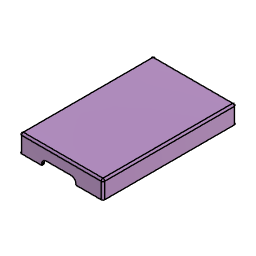
SlimCase-602030-FDM-Cover v3 (Autodesk Fusion 360 design; units mm, degrees)
Autodesk Fusion 360 part; units mm, degrees
sketch "Sketch1" plane through (0, 0, 0) normal (0, 0, 1) x (1, 0, 0)
  line L0 (11.7, 18.75) -> (-11.7, 18.75)
  line L1 (-11.7, 18.75) -> (-11.7, -18.75)
  line L2 (-11.7, -18.75) -> (11.7, -18.75)
  line L3 (11.7, -18.75) -> (11.7, 18.75)
  line L4 (11.7, 18.75) -> (-11.7, -18.75) construction
  line L5 (-11.7, 18.75) -> (11.7, -18.75) construction
  dimension "d1" = 23.4
  dimension "d2" = 37.5
  constraint horizontal L0
  constraint perpendicular L0 L1
  constraint parallel L0 L2
  constraint parallel L1 L3
  constraint coincident L4 origin
  constraint coincident L5 origin
  measures "d1" distance of L0.start L0.end
  measures "d2" distance of L0.end L1.end
extrude "Extrude1" add sketch "Sketch1" along normal blind 3.5
sketch "Sketch2" plane through (0, 0, 0) normal (0, 0, -1) x (1, 0, 0)
  line L0 (11.7, -18.75) -> (11.7, 18.75)
  line L1 (11.7, 18.75) -> (-11.7, 18.75)
  line L2 (-11.7, 18.75) -> (-11.7, -18.75)
  line L3 (-11.7, -18.75) -> (11.7, -18.75)
  line L4 (-10.1, -17.15) -> (10.1, -17.15)
  line L5 (10.1, -17.15) -> (10.1, 17.15)
  line L6 (10.1, 17.15) -> (-10.1, 17.15)
  line L7 (-10.1, 17.15) -> (-10.1, -17.15)
  line L8 (-10.1, -17.15) -> (10.1, 17.15) construction
  line L9 (10.1, -17.15) -> (-10.1, 17.15) construction
  line L10 (-11, -18.05) -> (11, -18.05)
  line L11 (11, -18.05) -> (11, 18.05)
  line L12 (11, 18.05) -> (-11, 18.05)
  line L13 (-11, 18.05) -> (-11, -18.05)
  line L14 (-11, -18.05) -> (11, 18.05) construction
  line L15 (11, -18.05) -> (-11, 18.05) construction
  dimension "d6" = 1.6
  dimension "d7" = 1.6
  dimension "d8" = 0.9
  dimension "d9" = 0.9
  constraint horizontal L4
  constraint perpendicular L4 L5
  constraint parallel L4 L6
  constraint parallel L5 L7
  constraint coincident L8 origin
  constraint coincident L9 origin
  constraint horizontal L10
  constraint perpendicular L10 L11
  constraint parallel L10 L12
  constraint parallel L11 L13
  constraint coincident L14 origin
  constraint coincident L15 origin
  measures "d6" distance of L3 L4
  measures "d7" distance of L2 L7
  measures "d8" distance of L4 L10
  measures "d9" distance of L7 L13
extrude "Extrude2" add sketch "Sketch2" along normal blind 1.5 contours L0 L1 L2 L3
sketch "Sketch3" plane through (0, 0, 0) normal (0, 0, -1) x (1, 0, 0)
  line L0 (-11, -18.05) -> (11, -18.05)
  line L1 (11, -18.05) -> (11, 18.05)
  line L2 (11, 18.05) -> (-11, 18.05)
  line L3 (-11, 18.05) -> (-11, -18.05)
  line L4 (-11, 18.05) -> (11, 18.05)
  line L5 (11, 18.05) -> (11, -18.05)
  line L6 (11, -18.05) -> (-11, -18.05)
  line L7 (-11, -18.05) -> (-11, 18.05)
  line L8 (10.4, 17.45) -> (-10.4, 17.45)
  line L9 (-10.4, 17.45) -> (-10.4, -17.45)
  line L10 (-10.4, -17.45) -> (10.4, -17.45)
  line L11 (10.4, -17.45) -> (10.4, 17.45)
  line L12 (10.4, 17.45) -> (-10.4, -17.45) construction
  line L13 (-10.4, 17.45) -> (10.4, -17.45) construction
  dimension "d12" = 0.6
  dimension "d13" = 0.6
  constraint horizontal L4
  constraint vertical L5
  constraint horizontal L6
  constraint vertical L7
  constraint coincident L0.end L1.start
  constraint coincident L2.end L3.start
  constraint horizontal L8
  constraint perpendicular L8 L9
  constraint parallel L8 L10
  constraint parallel L9 L11
  constraint coincident L12 origin
  constraint coincident L13 origin
  measures "d12" distance of L4 L8
  measures "d13" distance of L7 L9
extrude "Extrude3" cut sketch "Sketch3" against normal up to surface (2.5 mm away) contours L8 L9 L10 L11
sketch "Sketch4" plane through (0, -18.75, 0) normal (0, -1, 0) x (1, 0, 0)
  line L0 (11.7, -1.5) -> (11.7, 3.5)
  line L1 (11.7, 3.5) -> (-11.7, 3.5)
  line L2 (-11.7, 3.5) -> (-11.7, -1.5)
  line L3 (-11.7, -1.5) -> (11.7, -1.5)
  line L4 (-5.52, -1.5) -> (4.08, -1.5)
  line L5 (4.08, -1.5) -> (4.08, 0.2)
  line L6 (4.08, 0.2) -> (-5.52, 0.2)
  line L7 (-5.52, 0.2) -> (-5.52, -1.5)
  dimension "d16" = 6.18
  dimension "d17" = 9.6
  dimension "d18" = 1.7
  constraint horizontal L4
  constraint vertical L5
  constraint horizontal L6
  constraint vertical L7
  constraint coincident L3 L4.start
  measures "d16" distance of L2 L7
  measures "d17" distance of L5.end L6.end
  measures "d18" distance of L4.end L5.end
extrude "Extrude4" cut sketch "Sketch4" against normal up to surface (1.3 mm away) contours L3 L4 L5 L6 L7
fillet "Fillet1" radius 1.3 2 edges at (-5.52, -18.1, 0.2) (4.08, -18.1, 0.2)
sketch "Sketch5" plane through (11, 0, 0) normal (-1, 0, 0) x (0, -1, 0)
  line L0 (18.05, 0) -> (-18.05, 0)
  line L1 (-18.05, 0) -> (-18.05, -1.5)
  line L2 (-18.05, -1.5) -> (18.05, -1.5)
  line L3 (18.05, -1.5) -> (18.05, 0)
  line L4 (-18.05, 0) -> (18.05, -1.5) construction
  line L5 (18.05, 0) -> (-18.05, -1.5) construction
  line L6 (0, -0.75) -> (9.6098, -0.75) construction
  line L7 (6.5, -1) -> (-6.5, -1)
  line L8 (-6.5, -1) -> (-6.5, -0.5)
  line L9 (-6.5, -0.5) -> (6.5, -0.5)
  line L10 (6.5, -0.5) -> (6.5, -1)
  line L11 (6.5, -1) -> (-6.5, -0.5) construction
  line L12 (-6.5, -1) -> (6.5, -0.5) construction
  point P0 (0, -0.75)
  dimension "d23" = 13
  dimension "d24" = 0.5
  constraint coincident L0.end L1.start
  constraint coincident L2.end L3.start
  constraint coincident L0.start L3.end
  constraint coincident L1.end L2.start
  constraint midpoint L4 P0
  constraint parallel L2 L6
  constraint horizontal L7
  constraint perpendicular L7 L8
  constraint parallel L7 L9
  constraint parallel L8 L10
  constraint coincident L11 P0
  constraint coincident L12 P0
  constraint coincident P0 L6.start
  measures "d23" distance of L8.end L9.end
  measures "d24" distance of L7.start L9.end
extrude "Extrude5" add sketch "Sketch5" along normal blind 0.4 contours L7 L8 L9 L10
ref_plane "WorkPlane1" through (0, 0, 1) normal (-1, 0, 0) x (0, -1, 0)
mirror "Mirror1" about plane through (0, 0, 1) normal (-1, 0, 0) of "Extrude5"
fillet "Fillet2" radius 0.1 4 edges at (10.6, -6.5, -0.75) (10.6, 0, -1) (10.6, 0, -0.5) (10.6, 6.5, -0.75)
fillet "Fillet3" radius 0.1 4 edges at (-10.6, 0, -0.5) (-10.6, -6.5, -0.75) (-10.6, 0, -1) (-10.6, 6.5, -0.75)
fillet "Fillet4" radius 0.5 8 edges at (11.7, 0, 3.5) (0, -18.75, 3.5) (-11.7, 0, 3.5) (0, 18.75, 3.5) (-11.7, 18.75, 1) (-11.7, -18.75, 1) (11.7, 18.75, 1) (11.7, -18.75, 1)
fillet "Fillet5" radius 0.1 8 edges at (11, 0, -1) (11, 0, -0.5) (11, 6.5, -0.75) (11, -6.5, -0.75) (-11, 0, -1) (-11, -6.5, -0.75) (-11, 0, -0.5) (-11, 6.5, -0.75)
equation "d1 = 20.20 mm + 2 * ( case_thickness )"
equation "d2 = 34.3 mm + 2 * ( case_thickness )"
equation "d3 = lid_height"
equation "lid_height = 3.5 mm"
equation "d6 = case_thickness"
equation "d7 = case_thickness"
equation "d8 = case_thickness / 2 + 0.1 mm"
equation "d9 = case_thickness / 2 + 0.1 mm"
equation "d16 = 4.58 mm + case_thickness"
equation "d23 = 15 mm - 2 mm"
equation "case_thickness = 1.6 mm"
